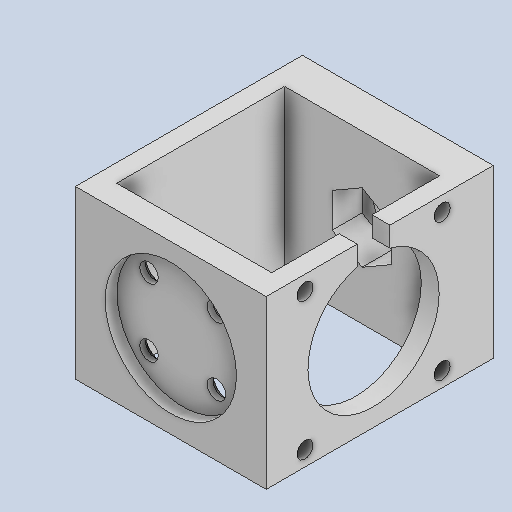
# Autodesk Inventor part: j6 motor mount
Saved by Autodesk Inventor 2025 (Build 290162000, 162)
## iProperties
Created: 2025-08-05
Part Number: j6 motor mount
Material: 一般
Document SubType Name: Modeling
Designer: gavin
Density: 1 g/cm^3
Appearance: 預設
Author: gavin
## iProperties of the stored document j6 motor mount_3D 列印.ipt
Created: 2025-08-05
Part Number: j6 motor mount_3D 列印
Material: 一般
Document SubType Name: Modeling
Designer: gavin
Density: 1 g/cm^3
Appearance: 預設
Author: gavin
Autodesk Inventor part; units mm, degrees
ref_plane "YZ Plane" through (0, 0, 0) normal (1, 0, 0) x (0, 1, 0)
ref_plane "XZ Plane" through (0, 0, 0) normal (0, 1, 0) x (-1, 0, 0)
sketch "草圖1" plane through (0, 0, 0) normal (1, 0, 0) x (0, 1, 0)
  line L0 (-14, 18) -> (14, 18)
  line L1 (14, 18) -> (14, -18)
  line L2 (14, -18) -> (-14, -18)
  line L3 (-14, -18) -> (-14, 18)
  line L4 (-14, 18) -> (14, -18) construction
  line L5 (14, 18) -> (-14, -18) construction
  line L6 (-11.5, 11.5) -> (11.5, 11.5) construction
  line L7 (11.5, 11.5) -> (11.5, -11.5) construction
  line L8 (11.5, -11.5) -> (-11.5, -11.5) construction
  line L9 (-11.5, -11.5) -> (-11.5, 11.5) construction
  line L10 (-11.5, 11.5) -> (11.5, -11.5) construction
  line L11 (11.5, 11.5) -> (-11.5, -11.5) construction
  circle A0 centre (11.5, 11.5) radius 1.35
  circle A1 centre (-11.5, 11.5) radius 1.35
  circle A2 centre (-11.5, -11.5) radius 1.35
  circle A3 centre (11.5, -11.5) radius 1.35
  circle A4 centre (0, 0) radius 11
  dimension "d0" = 28
  dimension "d1" = 36
  dimension "d2" = 23
  dimension "d3" = 23
  dimension "d4" = 2.7
  dimension "d7" = 360
  dimension "d9" = 22
  constraints: 24 end point, 5 centre point, 4 midpoint, 4 parallel, 2 coincident, 2 horizontal, 2 perpendicular, 9 other
  measures "d0" distance of L1.end L2.end
  measures "d1" distance of L0.end L1.end
  measures "d2" distance of L7.end L8.end
  measures "d3" distance of L6.end L7.end
  measures "d4" diameter of A0
  measures "d9" diameter of A4
extrude "擠出1" add sketch "草圖1" along normal blind 3
sketch "草圖2" plane through (0, 0, 0) normal (-1, 0, 0) x (0, 0, 1)
  line L0 (-18, -14) -> (-18, 14) projected
  line L1 (18, -14) -> (-18, -14) projected
  line L2 (18, 14) -> (18, -14) projected
  line L3 (-18, 14) -> (18, 14) projected
  circle A0 centre (0, 0) radius 11 projected
  circle A1 centre (-11.5, 11.5) radius 1.35 projected
  circle A2 centre (-11.5, -11.5) radius 1.35 projected
  circle A3 centre (11.5, -11.5) radius 1.35 projected
  circle A4 centre (11.5, 11.5) radius 1.35 projected
  line L4 (14.075, -14) -> (14.075, 14)
  line L5 (-14.075, -14) -> (-14.075, 14)
  dimension "d12" = 3.925
  dimension "d13" = 3.925
  constraints: 4 end point, 4 point on line, 2 perpendicular
  measures "d12" distance between parallel lines of L2 L4
  measures "d13" distance between parallel lines of L0 L5
extrude "擠出2" add sketch "草圖2" along normal blind 26 contours L0 L3 L5 L1 | L4 L3 L2 L1
sketch "草圖3" plane through (3, -14, 18) normal (0, 0, 1) x (1, 0, 0)
  line L0 (-29, 0) -> (0, 0) projected
  line L1 (0, 28) -> (0, 0) projected
  line L2 (-29, 28) -> (0, 28) projected
  line L3 (-29, 0) -> (-29, 28) projected
  circle A0 centre (-16, 14) radius 11
  line L4 (-3, 0) -> (-3, 28) projected
  line L5 (-3, 0) -> (-29, 0) projected
  line L6 (-29, 28) -> (-29, 0) projected
  line L7 (-3, 28) -> (-29, 28) projected
  point P0 (-3, 14)
  dimension "d16" = 22
  dimension "d17" = 13
  constraints: 1 centre point
  measures "d16" diameter of A0
  measures "d17" distance from line of A0.centre L4
extrude "擠出3" cut sketch "草圖3" against normal blind 2 contours A0
sketch "草圖4" plane through (3, 0, 0) normal (1, 0, 0) x (0, 0, -1)
  line L0 (-14.075, -14) -> (-14.075, 14) projected
  line L1 (18, -14) -> (18, 14) projected
  line L2 (18, 14) -> (-18, 14) projected
  line L3 (-18, 14) -> (-18, -14) projected
  line L4 (-18, -14) -> (18, -14) projected
  circle A0 centre (0, 0) radius 11 projected
  circle A1 centre (11.5, 11.5) radius 1.35 projected
  circle A2 centre (11.5, -11.5) radius 1.35 projected
  circle A3 centre (-11.5, -11.5) radius 1.35 projected
  circle A4 centre (-11.5, 11.5) radius 1.35 projected
  line L5 (-2.75, 14) -> (-2.75, 10.6507)
  line L6 (2.75, 14) -> (2.75, 10.6507)
  dimension "d20" = 5.5
  dimension "d21" = 2.75
  constraints: 4 end point, 2 point on circle, 2 point on line, 2 vertical
  measures "d20" distance between parallel lines of L6 L5
  measures "d21" distance from line of point (0, 0) L6
extrude "擠出4" cut sketch "草圖4" against normal up to surface (3 mm away) contours L2 L6 A0 L5
sketch "草圖5" plane through (-26, 0, 0) normal (-1, 0, 0) x (0, 0, 1)
  line L0 (-18, -14) -> (-14.075, -14) projected
  line L1 (-14.075, -14) -> (-14.075, 14) projected
  line L2 (-14.075, 14) -> (-18, 14) projected
  line L3 (-18, 14) -> (-18, -14) projected
  line L4 (16, 11) -> (16, -11) projected
  line L5 (18, 14) -> (14.075, 14) projected
  line L6 (14.075, 14) -> (14.075, -14) projected
  line L7 (14.075, -14) -> (18, -14) projected
  line L8 (18, -14) -> (18, 14) projected
  line L9 (-18, -14) -> (-18, 14) projected
  line L10 (-18, -14) -> (18, -14)
  line L11 (18, -14) -> (18, 14)
  line L12 (18, 14) -> (-18, 14)
  line L13 (-18, 14) -> (-18, -14)
  point P0 (0, 0)
  constraints: 8 end point, 2 parallel, 1 horizontal, 1 perpendicular
extrude "擠出5" add sketch "草圖5" along normal blind 3
sketch "草圖6" plane through (3, -14, -18) normal (0, 0, -1) x (-1, 0, 0)
  line L0 (32, 28) -> (0, 28) projected
  line L1 (0, 0) -> (0, 28) projected
  line L2 (0, 0) -> (32, 0) projected
  line L3 (32, 28) -> (32, 0) projected
  point P0 (3, 14)
extrude "擠出6" add sketch "草圖6" along normal blind 2.075
sketch "草圖7" plane through (0, -14, -14.075) normal (0, 0, 1) x (1, 0, 0)
  circle A0 centre (-13, 14) radius 11 projected
  line L0 (-13, 19.7735) -> (-8, 16.8868)
  line L1 (-8, 16.8868) -> (-8, 11.1132)
  line L2 (-8, 11.1132) -> (-13, 8.2265)
  line L3 (-13, 8.2265) -> (-18, 11.1132)
  line L4 (-18, 11.1132) -> (-18, 16.8868)
  line L5 (-18, 16.8868) -> (-13, 19.7735)
  point P0 (0, 14)
  dimension "d28" = 10
  constraints: 12 end point, 1 coincident, 13 other
  measures "d28" distance between parallel lines of L1 L4
extrude "擠出7" cut sketch "草圖7" against normal blind 5 contours L0 L1 L2 L3 L4 L5
sketch "草圖8" plane through (-13, 0, 16) normal (0, 0, 1) x (1, 0, 0)
  circle A0 centre (0, 0) radius 11 projected
  circle A1 centre (0, 0) radius 8 construction
  line L0 (0, 0) -> (-5.6569, 5.6569) construction
  line L1 (0, 0) -> (8, 0) construction
  circle A2 centre (-5.6569, 5.6569) radius 1.55
  circle A3 centre (-5.6569, -5.6569) radius 1.55
  circle A4 centre (5.6569, -5.6569) radius 1.55
  circle A5 centre (5.6569, 5.6569) radius 1.55
  point P0 (13, 0)
  dimension "d31" = 16
  dimension "d32" = 135
  dimension "d33" = 3.1
  dimension "d36" = 360
  constraints: 4 centre point, 4 end point, 2 coincident, 1 equal length, 1 horizontal, 12 other
  measures "d32" angle of L1 L0
  measures "d33" diameter of A2
extrude "擠出8" cut sketch "草圖8" against normal up to surface (1.925 mm away) contours A2 | A3 | A4 | A5
chamfer "倒角1" distance 0.95 angle 45 4 edges at (-20.2069, 5.6569, 14.075) (-20.2069, -5.6569, 14.075) (-8.8931, 5.6569, 14.075) (-8.8931, -5.6569, 14.075)
sketch "草圖9" plane through (0, -14, -19.075) normal (0, 0, 1) x (1, 0, 0)
  circle A0 centre (-13, 14) radius 11 projected
  circle A1 centre (-13, 14) radius 3.1
  point P0 (0, 14)
  dimension "d43" = 6.2
  constraints: 1 centre point, 1 coincident
  measures "d43" diameter of A1
extrude "擠出9" cut sketch "草圖9" against normal through all contours A1
ref_plane "工作平面1" through (-32.62, 0.0998, -6) normal (0, 1, 0) x (1, 0, 0)
sketch "草圖10" plane through (-32.62, 0.0998, -6) normal (0, 1, 0) x (1, 0, 0)
  line L0 (-7.96, 0) -> (0, 0) projected
  line L1 (0, 0) -> (0, 4) projected
  line L2 (0, 4) -> (-9.8, 4) projected
  line L3 (-9.8, -8.94) -> (-9.8, 4) projected
  line L4 (-9.8, -8.94) -> (0, -8.94) projected
  line L5 (0, -8.94) -> (0, -4.94) projected
  line L6 (0, -4.94) -> (-7.96, -4.94) projected
  line L7 (-7.96, -4.94) -> (-7.96, 0) projected
  line L8 (35.62, -8.75) -> (32.62, -8.75) projected
  line L9 (32.62, -8.75) -> (32.62, -20.075) projected
  line L10 (32.62, -20.075) -> (6.62, -20.075) projected
  line L11 (6.62, -20.075) -> (6.62, 8.075) projected
  line L12 (32.62, 8.075) -> (6.62, 8.075) projected
  line L13 (32.62, 8.075) -> (32.62, -3.25) projected
  line L14 (32.62, -3.25) -> (35.62, -3.25) projected
  line L15 (35.62, -3.25) -> (35.62, 14.075) projected
  line L16 (3.62, 14.075) -> (35.62, 14.075) projected
  line L17 (3.62, -24) -> (3.62, 14.075) projected
  line L18 (3.62, -24) -> (35.62, -24) projected
  line L19 (35.62, -8.75) -> (35.62, -24) projected
  line L20 (3.62, -3.72) -> (-5.88, -3.72)
  line L21 (-5.88, -3.72) -> (-5.88, -1.22)
  line L22 (-5.88, -1.22) -> (3.62, -1.22)
  point P0 (32.62, -6)
  dimension "d46" = 2.5
  dimension "d47" = 4.94
  dimension "d48" = 1.22
  dimension "d52" = 9.5
  constraints: 6 end point, 2 perpendicular, 2 point on line, 1 horizontal
  measures "d46" distance of L20.end L21.end
  measures "d47" distance of L6.end L0.start
  measures "d48" distance between parallel lines of L0 L22
  measures "d52" distance of L21.end L22.end
extrude "擠出10" add sketch "草圖10" against normal up to surface (6.1003 mm away) contours L20 L21 L22 L17
fillet "圓角1" radius 2 4 edges at (-29, -2.9503, -2.28) (-29, 0.0998, -3.53) (-29, -2.9503, -4.78) (-29, -6.0005, -3.53)
equation "\"d12\" = d13"
equation "\"d21\" = 0.5 * d20"
